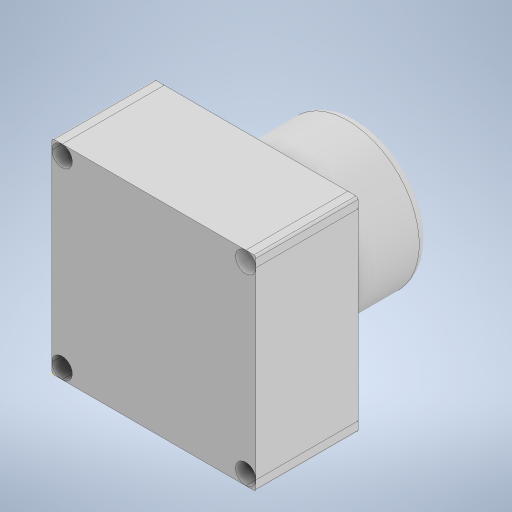
# Autodesk Inventor part: Tarea1jrsr
Saved by Autodesk Inventor 2024 (Build 280153000, 153)
## iProperties
Created: 2024-02-06
Part Number: Tarea1jrsr
Material: Generic
Document SubType Name: Modeling
Designer: joser
Density: 1 g/cm^3
Appearance: Default
Author: joser
Autodesk Inventor part; units mm, degrees
ref_plane "YZ Plane" through (0, 0, 0) normal (1, 0, 0) x (0, 1, 0)
ref_plane "XZ Plane" through (0, 0, 0) normal (0, 1, 0) x (-1, 0, 0)
ref_plane "XY Plane" through (0, 0, 0) normal (0, 0, 1) x (1, 0, 0)
sketch "Sketch1" plane through (0, 0, 0) normal (0, 0, 1) x (1, 0, 0)
  line L0 (0, 0) -> (100, 0)
  line L1 (100, 0) -> (100, 100)
  line L2 (100, 100) -> (0, 100)
  line L3 (0, 100) -> (0, 0)
  dimension "d0" = 100
  dimension "d1" = 100
  constraints: 8 end point, 2 parallel, 1 horizontal, 1 perpendicular
  measures "d0" distance of L2.end L1.end
  measures "d1" distance of L1.end L0.end
extrude "Extrusion1" add sketch "Sketch1" along normal blind 50
sketch "Sketch2" plane through (0, 0, 50) normal (0, 0, 1) x (1, 0, 0)
  point P0 (0, 0)
sketch "Sketch5" plane through (0, 0, 50) normal (0, 0, 1) x (1, 0, 0)
  line L0 (5, 5) -> (95, 95) construction
  line L1 (95, 5) -> (5, 95) construction
  circle A0 centre (5, 95) radius 5
  line L2 (0, 100) -> (0, 0) projected
  circle A1 centre (95, 95) radius 5
  line L3 (100, 100) -> (0, 100) projected
  circle A2 centre (95, 5) radius 5
  circle A3 centre (5, 5) radius 5
  point P0 (50, 50)
  dimension "d11" = 90
  dimension "d12" = 90
  constraints: 4 centre point, 4 coincident, 4 end point, 2 midpoint, 2 tangent
  measures "d11" distance of L1.end L0.end
  measures "d12" distance of L0.end L1.start
extrude "Extrusion2" cut sketch "Sketch5" against normal blind 50 contours A0 | A3 | A1 | A2
fillet "Fillet1" radius 1 1 edges at (0, 100, 25)
fillet "Fillet2" radius 1 1 edges at (100, 100, 25)
fillet "Fillet3" radius 1 1 edges at (0, 0, 25)
fillet "Fillet4" radius 1 1 edges at (100, 0, 25)
sketch "Sketch6" plane through (0, 0, 0) normal (0, 0, -1) x (-1, 0, 0)
  line L0 (-15, 15) -> (-85, 85) construction
  line L1 (-85, 15) -> (-15, 85) construction
  circle A0 centre (-50, 50) radius 35
  point P0 (0, 0)
  dimension "d20" = 70
  dimension "d21" = 70
  constraints: 4 end point, 2 midpoint, 1 centre point, 1 coincident
  measures "d20" distance of L0.end L1.end
  measures "d21" distance of L1.start L0.end
extrude "Extrusion3" add sketch "Sketch6" along normal blind 50
sketch "Sketch7" plane through (50, 50, -50) normal (0, 0, -1) x (-1, 0, 0)
  circle A0 centre (0, 0) radius 25
  point P0 (50, -50)
  dimension "d24" = 50
  constraints: 1 centre point
  measures "d24" diameter of A0
extrude "Extrusion4" cut sketch "Sketch7" against normal blind 30
fillet "Fillet5" radius 5 1 edges at (85, 50, -50)
thread "Thread1" size "M50x4" class "6H" standard "ANSI Metric M Profile" full length
body "Solid1"
